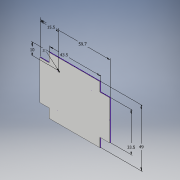
# Autodesk Inventor part: Protoboard
Saved by Autodesk Inventor 2019.3 (Build 233278000, 278)
## iProperties
Created: 2019-06-06
Part Number: Protoboard
Material: Generic
Document SubType Name: Modeling
Designer: Frienddo
Density: 1 g/cm^3
Appearance: Default
Author: Frienddo
Autodesk Inventor part; units mm, degrees
ref_plane "YZ Plane" through (0, 0, 0) normal (1, 0, 0) x (0, 1, 0)
ref_plane "XZ Plane" through (0, 0, 0) normal (0, 1, 0) x (-1, 0, 0)
ref_plane "XY Plane" through (0, 0, 0) normal (0, 0, 1) x (1, 0, 0)
sketch "Sketch1" plane through (0, 0, 0) normal (0, 0, 1) x (1, 0, 0)
  line L0 (0, 0) -> (-29.85, 0)
  line L1 (-29.85, 0) -> (-29.85, 16.75)
  line L2 (-29.85, 16.75) -> (-21.75, 16.75)
  line L3 (-21.75, 16.75) -> (-21.75, 24.5)
  line L4 (-21.75, 24.5) -> (0, 24.5)
  line L5 (0, 24.5) -> (0, 0)
  circle A0 centre (-14.35, 14.5) radius 1.5
  line L6 (0, 0) -> (29.85, 0)
  line L7 (29.85, 0) -> (29.85, 16.75)
  line L8 (29.85, 16.75) -> (21.75, 16.75)
  line L9 (21.75, 16.75) -> (21.75, 24.5)
  line L10 (21.75, 24.5) -> (0, 24.5)
  circle A1 centre (14.35, 14.5) radius 1.5
  line L11 (-29.85, 0) -> (-29.85, -16.75)
  line L12 (-29.85, -16.75) -> (-21.75, -16.75)
  line L13 (-21.75, -16.75) -> (-21.75, -24.5)
  line L14 (-21.75, -24.5) -> (0, -24.5)
  line L15 (0, -24.5) -> (0, 0)
  circle A2 centre (-14.35, -14.5) radius 1.5
  line L16 (29.85, 0) -> (29.85, -16.75)
  line L17 (29.85, -16.75) -> (21.75, -16.75)
  line L18 (21.75, -16.75) -> (21.75, -24.5)
  line L19 (21.75, -24.5) -> (0, -24.5)
  circle A3 centre (14.35, -14.5) radius 1.5
  dimension "d0" = 15.5
  dimension "d1" = 10
  dimension "d2" = 43.5
  dimension "d3" = 59.7
  dimension "d4" = 49
  dimension "d5" = 33.5
  dimension "d6" = 3
  constraints: 40 end point, 14 symmetric about line, 5 perpendicular, 4 centre point, 1 horizontal, 3 other
  measures "d0" distance from line of L1 A0.centre
  measures "d1" distance from line of L4 A0.centre
  measures "d2" distance between parallel lines of L3 L9
  measures "d3" distance between parallel lines of L7 L1
  measures "d4" distance between parallel lines of L19 L10
  measures "d5" distance between parallel lines of L17 L8
  measures "d6" diameter of A0
extrude "Extrusion3" add sketch "Sketch1" along normal blind 0.5 contours L15 L14 L13 L12 L11 L0 | L0 L1 L2 L3 L4 L5 | L5 L10 L9 L8 L7 L6 | L6 L16 L17 L18 L19 L15 | A0 | A1 | A2 | A3
sketch "Sketch2" plane through (0, 0, 0) normal (0, 0, -1) x (-1, 0, 0)
  circle A0 centre (14.35, 14.5) radius 1.5 projected
  circle A1 centre (14.35, 14.5) radius 1
  circle A2 centre (14.35, -14.5) radius 1.5 projected
  circle A3 centre (-14.35, -14.5) radius 1.5 projected
  circle A4 centre (-14.35, 14.5) radius 1.5 projected
  circle A5 centre (14.35, -14.5) radius 1
  circle A6 centre (-14.35, -14.5) radius 1
  circle A7 centre (-14.35, 14.5) radius 1
  point P0 (0, 0)
  dimension "d13" = 0.5
  dimension "d14" = 0.5
  dimension "d15" = 0.5
  dimension "d16" = 0.5
  constraints: 4 centre point
  measures "d13" radial gap between concentric circles of A0 A1
  measures "d14" radial gap between concentric circles of A2 A5
  measures "d15" radial gap between concentric circles of A3 A6
  measures "d16" radial gap between concentric circles of A4 A7
extrude "Extrusion4" add sketch "Sketch2" along normal blind 6 contours A1 | A5 | A6 | A7
body "Solid1"
body "Solid3"
